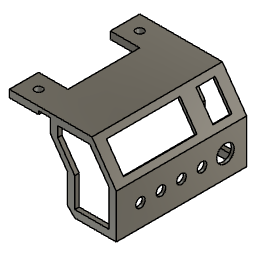
종합 스위치 브라켓 (Autodesk Fusion 360 design; units mm, degrees)
Autodesk Fusion 360 part; units mm, degrees
note: some values were not read from the file. Set by a fixed rule: which sketch regions a step uses.
sketch "스케치1" plane through (0, 0, 0) normal (0, 1, 0) x (1, 0, 0)
  line L0 (0, 0) -> (0, -30)
  line L1 (0, -30) -> (-16.6337, -53.7554)
  line L2 (0, -30) -> (29, -30) construction
  line L3 (0, 0) -> (-2, 0)
  line L4 (-16.6337, -53.7554) -> (-18.272, -52.6083)
  line L5 (-18.272, -52.6083) -> (-2, -29.3694)
  line L6 (-2, 0) -> (-2, -29.3694)
  line L7 (0, 0) -> (-73, 0)
  line L8 (-16.6337, -53.7554) -> (-73, -53.7554)
  line L9 (-18.272, -52.6083) -> (-17.1249, -50.97)
  line L10 (-73, -53.7554) -> (-73, -48.7554)
  line L11 (-73, -48.7554) -> (-53, -48.7554)
  line L12 (-53, -48.7554) -> (-53, -53.7554)
  line L13 (-17.1249, -50.97) -> (-53, -50.97)
  line L14 (-53, -50.97) -> (-45, -50.97)
  line L15 (-45, -50.97) -> (-45, 0)
  dimension "d1" = 30
  dimension "d2" = 125
  dimension "d3" = 29
  dimension "d4" = 2
  dimension "d7" = 73
  dimension "d8" = 2
  dimension "d9" = 5
  dimension "d10" = 20
  dimension "d11" = 8
  constraint coincident L0.start L3.start
  constraint vertical L0
  constraint horizontal L2
  constraint perpendicular L0 L3
  constraint perpendicular L1 L4
  constraint perpendicular L4 L5
  constraint perpendicular L3 L6
  constraint perpendicular L6 L7
  constraint parallel L7 L8
  constraint perpendicular L4 L9
  constraint perpendicular L8 L10
  constraint perpendicular L10 L11
  constraint coincident L8 L12.end
  constraint perpendicular L8 L12
  constraint coincident L12 L13.end
  constraint perpendicular L12 L13
  constraint perpendicular L12 L14
  constraint coincident L7 L15.end
  constraint perpendicular L7 L15
  measures "d1" distance of L0.start L0.end
  measures "d2" angle of L1 L2
  measures "d3" distance of L0.end L1.end
  measures "d4" distance of L1.end L4.end
  measures "d7" distance of L0.start L7.end
  measures "d8" distance of L4.end L9.end
  measures "d9" distance of L8.end L10.end
  measures "d10" distance of L10.end L11.end
  measures "d11" distance of L13.end L14.end
extrude "돌출1" add sketch "스케치1" along normal blind 88.975 contours L0 L1 L3 L4 L5 L6 L7 L9 | L4 L5 L8 L9 L12 L13 L14 | L8 L10 L11 L12
extrude "돌출2" add sketch "스케치1" along normal blind 3 contours L5 L6 L7 L13 L15
sketch "스케치2" plane through (0, 88.975, 0) normal (0, 1, 0) x (-1, 0, 0)
  line L0 (0, 0) -> (2, 0)
  line L1 (2, 0) -> (2, 29.3694)
  line L2 (2, 29.3694) -> (17.1249, 50.97)
  line L3 (17.1249, 50.97) -> (53, 50.97)
  line L4 (53, 50.97) -> (53, 48.7554)
  line L5 (53, 48.7554) -> (73, 48.7554)
  line L6 (73, 48.7554) -> (73, 53.7554)
  line L7 (73, 53.7554) -> (16.6337, 53.7554)
  line L8 (16.6337, 53.7554) -> (0, 30)
  line L9 (0, 30) -> (0, 0)
  line L10 (53, 50.97) -> (45, 50.97)
  line L11 (45, 50.97) -> (45, 0)
  line L12 (45, 0) -> (2, 0)
  dimension "d14" = 8
  constraint coincident L3.end L4.start
  constraint perpendicular L4 L10
  constraint perpendicular L10 L11
  constraint coincident L0.end L1.start
  constraint perpendicular L1 L12
  measures "d14" distance of L3.end L10.end
extrude "돌출3" add sketch "스케치2" against normal blind 3 contours L1 L2 L3 L11 L12
sketch "스케치3" plane through (0, 0, 0) normal (1, 0, 0) x (0, 1, 0)
  line L0 (0, 30) -> (0, 0)
  line L1 (0, 0) -> (88.975, 0)
  line L2 (88.975, 0) -> (88.975, 30)
  line L3 (88.975, 30) -> (0, 30)
  line L4 (86.4875, 30) -> (2.4875, 30)
  line L5 (2.4875, 30) -> (2.4875, 0)
  line L6 (2.4875, 0) -> (86.4875, 0)
  line L7 (86.4875, 0) -> (86.4875, 30)
  line L8 (86.4875, 30) -> (2.4875, 0) construction
  line L9 (2.4875, 30) -> (86.4875, 0) construction
  line L10 (2.4875, 15) -> (16.4875, 15)
  line L11 (16.4875, 15) -> (30.4875, 15)
  line L12 (30.4875, 15) -> (44.4875, 15)
  line L13 (44.4875, 15) -> (58.4875, 15)
  line L14 (58.4875, 15) -> (74.4875, 15)
  line L15 (74.4875, 15) -> (86.4875, 15)
  circle A0 centre (16.4875, 15) radius 3.25
  circle A1 centre (30.4875, 15) radius 3.25
  circle A2 centre (44.4875, 15) radius 3.25
  circle A3 centre (58.4875, 15) radius 3.25
  circle A4 centre (74.4875, 15) radius 6
  circle A5 centre (16.4875, 15) radius 6
  point P0 (44.4875, 15)
  dimension "d45" = 84
  dimension "d46" = 14
  dimension "d47" = 14
  dimension "d48" = 14
  dimension "d49" = 14
  dimension "d50" = 16
  dimension "d51" = 6.5
  dimension "d52" = 6.5
  dimension "d53" = 6.5
  dimension "d54" = 6.5
  dimension "d55" = 12
  dimension "d56" = 12
  constraint horizontal L4
  constraint perpendicular L4 L5
  constraint parallel L4 L6
  constraint parallel L5 L7
  constraint coincident L8 P0
  constraint coincident L9 P0
  constraint midpoint L5 L10.start
  constraint perpendicular L5 L10
  constraint perpendicular L5 L11
  constraint parallel L10 L12
  constraint coincident P0 L12.end
  constraint parallel L12 L13
  constraint parallel L13 L14
  constraint midpoint L7 L15.end
  constraint coincident L10.end L11.start
  constraint coincident L11.end L12.start
  constraint coincident L13.end L14.start
  constraint coincident L14.end L15.start
  constraint concentric A0 A5
  measures "d45" distance of L5.end L6.end
  measures "d46" distance of L10.start L10.end
  measures "d47" distance of L10.end L11.end
  measures "d48" distance of L11.end P0
  measures "d49" distance of P0 L13.end
  measures "d50" distance of L13.end L14.end
  measures "d51" diameter of A0
  measures "d52" diameter of A1
  measures "d53" diameter of A2
  measures "d54" diameter of A3
  measures "d55" diameter of A4
  measures "d56" diameter of A5
extrude "돌출4" cut sketch "스케치3" against normal blind 3 contours L14 L15 A4 | L14 L15 A4 | L10 L11 A0 | L10 L11 A0 | L11 L12 A1 | L11 L12 A1 | L13 L14 A3 | L13 L14 A3 | L12 L13 A2 | L12 L13 A2
sketch "스케치4" plane through (14.0954, 0, 9.8697) normal (0.819152, 0, 0.573576) x (0, 1, 0)
  line L0 (0, 53.5746) -> (0, 24.5746)
  line L1 (0, 24.5746) -> (88.975, 24.5746)
  line L2 (88.975, 24.5746) -> (88.975, 53.5746)
  line L3 (88.975, 53.5746) -> (0, 53.5746)
  line L4 (0, 39.0746) -> (32.5, 39.0746)
  line L5 (7.4, 28.9746) -> (57.6, 28.9746)
  line L6 (57.6, 28.9746) -> (57.6, 49.1746)
  line L7 (57.6, 49.1746) -> (7.4, 49.1746)
  line L8 (7.4, 49.1746) -> (7.4, 28.9746)
  line L9 (7.4, 28.9746) -> (57.6, 49.1746) construction
  line L10 (57.6, 28.9746) -> (7.4, 49.1746) construction
  line L11 (88.975, 39.0746) -> (75, 39.0746)
  line L12 (68.525, 49.0746) -> (81.475, 49.0746)
  line L13 (81.475, 49.0746) -> (81.475, 29.0746)
  line L14 (81.475, 29.0746) -> (68.525, 29.0746)
  line L15 (68.525, 29.0746) -> (68.525, 49.0746)
  line L16 (68.525, 49.0746) -> (81.475, 29.0746) construction
  line L17 (81.475, 49.0746) -> (68.525, 29.0746) construction
  point P0 (32.5, 39.0746)
  point P1 (75, 39.0746)
  dimension "d37" = 32.5
  dimension "d38" = 50.2
  dimension "d39" = 20.2
  dimension "d40" = 13.975
  dimension "d41" = 12.95
  dimension "d42" = 20
  constraint midpoint L0 L4.start
  constraint perpendicular L0 L4
  constraint horizontal L5
  constraint perpendicular L5 L6
  constraint parallel L5 L7
  constraint parallel L6 L8
  constraint coincident L9 P0
  constraint coincident L10 P0
  constraint coincident P0 L4.end
  constraint midpoint L2 L11.start
  constraint perpendicular L2 L11
  constraint horizontal L12
  constraint perpendicular L12 L13
  constraint parallel L12 L14
  constraint parallel L13 L15
  constraint coincident L16 P1
  constraint coincident L17 P1
  constraint coincident P1 L11.end
  measures "d37" distance of L4.start P0
  measures "d38" distance of L6.end L7.end
  measures "d39" distance of L5.end L6.end
  measures "d40" distance of L11.start P1
  measures "d41" distance of L13.end L14.end
  measures "d42" distance of L12.end L13.end
extrude "돌출5" cut sketch "스케치4" against normal blind 3 contours L5 L6 L7 L8 | L12 L13 L14 L15
sketch "스케치5" plane through (0, 88.975, 0) normal (0, 1, 0) x (-1, 0, 0)
  line L0 (0, 0) -> (45, 0)
  line L1 (45, 0) -> (45, 50.97)
  line L2 (45, 50.97) -> (53, 50.97)
  line L3 (53, 50.97) -> (53, 48.7554)
  line L4 (53, 48.7554) -> (73, 48.7554)
  line L5 (73, 48.7554) -> (73, 53.7554)
  line L6 (73, 53.7554) -> (16.6337, 53.7554)
  line L7 (16.6337, 53.7554) -> (0, 30)
  line L8 (0, 30) -> (0, 0)
  line L9 (0, 30) -> (5, 30)
  line L10 (5, 0) -> (5, 5)
  line L11 (5, 5) -> (5, 30)
  line L12 (5, 5) -> (40, 5)
  line L13 (5, 30) -> (21.6337, 53.7554)
  line L14 (5, 30) -> (5, 25)
  line L15 (5, 25) -> (45, 25)
  line L16 (45, 53.7554) -> (45, 48.7554)
  line L17 (45, 48.7554) -> (28.3663, 25)
  line L18 (28.3663, 25) -> (28.3663, 0)
  line L19 (28.3663, 5) -> (33.3663, 5)
  line L20 (33.3663, 5) -> (33.3663, 0)
  line L21 (33.3663, 5) -> (33.3663, 25)
  line L22 (45, 48.7554) -> (50, 48.7554)
  line L23 (50, 48.7554) -> (33.3663, 25)
  line L24 (45, 48.7554) -> (18.1327, 48.7554)
  line L25 (45, 53.7554) -> (40, 53.7554)
  line L26 (40, 53.7554) -> (40, 34.4739)
  line L27 (40, 34.4739) -> (45, 34.4739)
  line L28 (45, 34.4739) -> (45, 53.7554)
  line L29 (33.3663, 5) -> (28.3663, 0)
  dimension "d57" = 5
  dimension "d58" = 5
  dimension "d59" = 35
  dimension "d60" = 29
  dimension "d61" = 5
  dimension "d62" = 5
  dimension "d63" = 29
  dimension "d64" = 5
  dimension "d65" = 5
  dimension "d66" = 5
  constraint coincident L7.end L8.start
  constraint perpendicular L8 L9
  constraint coincident L0 L10.start
  constraint perpendicular L0 L10
  constraint perpendicular L1 L12
  constraint coincident L6 L13.end
  constraint perpendicular L9 L14
  constraint coincident L1 L15.end
  constraint perpendicular L1 L15
  constraint coincident L6 L16.start
  constraint perpendicular L2 L16
  constraint coincident L15 L17.end
  constraint coincident L0 L18.end
  constraint perpendicular L0 L18
  constraint coincident L18 L19.start
  constraint coincident L12 L19.start
  constraint perpendicular L18 L19
  constraint coincident L0 L20.end
  constraint perpendicular L0 L20
  constraint coincident L15 L21.end
  constraint perpendicular L15 L21
  constraint perpendicular L16 L22
  constraint coincident L13 L24.end
  constraint perpendicular L1 L24
  constraint horizontal L25
  constraint vertical L26
  constraint horizontal L27
  constraint vertical L28
  constraint coincident L23 L26.end
  measures "d57" distance of L7.end L9.end
  measures "d58" distance of L10.start L10.end
  measures "d59" distance of L10.end L12.end
  measures "d60" distance of L9.end L13.end
  measures "d61" distance of L9.end L14.end
  measures "d62" distance of L16.start L16.end
  measures "d63" distance of L16.end L17.end
  measures "d64" distance of L19.start L19.end
  measures "d65" distance of L16.end L22.end
  measures "d66" distance of L16.start L25.end
extrude "돌출6" cut sketch "스케치5" against normal blind 88.975 contours L0 L20 L29 | L11 L12 L15 L18 | L11 L13 L14 L15 L17 L24 L26 | L0 L1 L15 L20 L21 | L1 L15 L23 L27 | L1 L23 L27 L28
sketch "스케치6" plane through (0, 0, 53.7554) normal (0, 0, 1) x (-1, 0, 0)
  line L0 (73, 0) -> (16.6337, 0)
  line L1 (16.6337, 0) -> (16.6337, -88.975)
  line L2 (16.6337, -88.975) -> (73, -88.975)
  line L3 (73, -88.975) -> (73, 0)
  line L4 (73, 0) -> (53, 0)
  line L5 (53, 0) -> (53, -88.975)
  line L6 (53, -88.975) -> (73, -88.975)
  line L7 (73, -88.975) -> (73, 0)
  line L8 (73, 0) -> (53, 0)
  line L9 (53, 0) -> (53, -20)
  line L10 (53, -20) -> (73, -20)
  line L11 (73, -20) -> (73, 0)
  line L12 (73, -88.975) -> (53, -88.975)
  line L13 (53, -88.975) -> (53, -68.975)
  line L14 (53, -68.975) -> (73, -68.975)
  line L15 (73, -68.975) -> (73, -88.975)
  circle A0 centre (63, -10) radius 2.65
  circle A1 centre (63, -78.975) radius 2.65
  dimension "d69" = 20
  dimension "d70" = 20
  dimension "d71" = 20
  dimension "d72" = 5.3
  dimension "d73" = 5.3
  constraint horizontal L4
  constraint vertical L5
  constraint horizontal L6
  constraint vertical L7
  constraint coincident L2 L5.end
  constraint coincident L0.start L3.end
  constraint horizontal L8
  constraint vertical L9
  constraint horizontal L10
  constraint vertical L11
  constraint horizontal L12
  constraint vertical L13
  constraint horizontal L14
  constraint vertical L15
  constraint coincident L2.end L3.start
  measures "d69" distance of L0.start L4.end
  measures "d70" distance of L0.start L10.end
  measures "d71" distance of L2.end L14.end
  measures "d72" diameter of A0
  measures "d73" diameter of A1
extrude "돌출7" cut sketch "스케치6" against normal blind 5 contours L3 L5 L7 L10 L14 | A0 | A1
